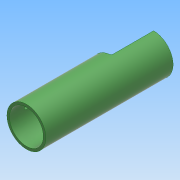
# Autodesk Inventor part: Pancake_Lower Pipe
Saved by Autodesk Inventor 2018.1 (Build 221171000, 171)
## iProperties
Created: 2019-02-21
Part Number: Pancake_Lower Pipe
Material: PVC-Piping
Document SubType Name: Modeling
Designer: James
Density: 1.4 g/cm^3
Appearance: Smooth - Dark Forest Green
Author: James
Autodesk Inventor part; units mm, degrees
ref_plane "YZ Plane" through (0, 0, 0) normal (1, 0, 0) x (0, 1, 0)
ref_plane "XZ Plane" through (0, 0, 0) normal (0, 1, 0) x (-1, 0, 0)
ref_plane "XY Plane" through (0, 0, 0) normal (0, 0, 1) x (1, 0, 0)
sketch "Sketch1" plane through (0, 0, 0) normal (0, 1, 0) x (-1, 0, 0)
  circle A0 centre (0, 0) radius 20
  circle A1 centre (0, 0) radius 23
  dimension "d0" = 40
  dimension "d1" = 3
  constraints: 2 centre point, 2 coincident
  measures "d0" diameter of A0
  measures "d1" radial gap between concentric circles of A0 A1
extrude "Extrusion1" add sketch "Sketch1" along normal mid plane 150
sketch "Sketch2" plane through (0, 0, 0) normal (1, 0, 0) x (0, 1, 0)
  line L0 (-105, 0) -> (105, 0) projected
  line L1 (-75, 23) -> (-75, -23) projected
  point P0 (0, 0)
  point P1 (5, 0)
  point P2 (-55, 0)
  dimension "d4" = 60
  dimension "d5" = 20
  constraints: 1 horizontal alignment, 1 point on line
  measures "d4" distance of point (-55, 0) point (5, 0)
  measures "d5" distance from line of L1 point (-55, 0)
hole "Hole1" at (0, 5, 0) at (0, -55, 0) direction (-1, 0, 0) diameter 4.5 end through all clearance for "Socket Head Cap Screw" size "M4" standard "Ansi Metric M Profile"
sketch "Sketch3" plane through (0, 0, 0) normal (0, 0, 1) x (1, 0, 0)
  line L0 (23, 75) -> (-23, 75) projected
  line L1 (-23, -75) -> (-23, 75) projected
  line L2 (-23, 75) -> (0, 75)
  line L3 (0, 75) -> (0, 25)
  line L4 (0, 25) -> (-23, 25)
  line L5 (-23, 25) -> (-23, 75)
  point P0 (0, 0)
  dimension "d13" = 50
  dimension "d14" = 23
  dimension "d15" = 46
  constraints: 8 end point, 2 parallel, 1 horizontal, 1 perpendicular
  measures "d13" distance of L2.end L3.end
  measures "d14" distance of L3.end L4.end
  measures "d15" distance of L0.start L0.end
extrude "Extrusion2" cut sketch "Sketch3" along normal through all both and the other way through all
fillet "Fillet1" radius 2 2 edges at (0, 25, 21.5) (0, 25, -21.5)
equation "\"d14\" = 0.5 * d15"
body "Solid1"
